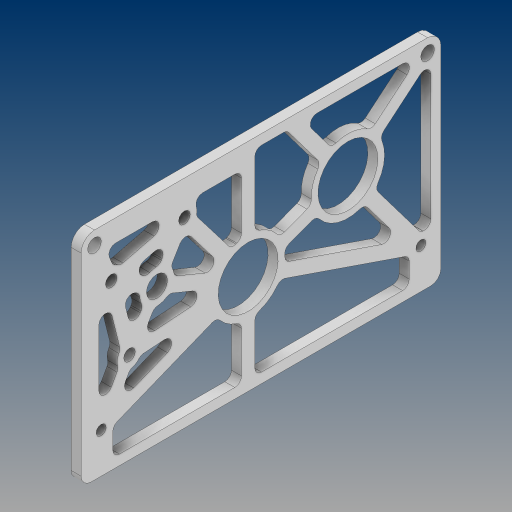
# Autodesk Inventor part: Intake Pivot Gearbox
Saved by Autodesk Inventor 2024.3 (Build 283343000, 343)
## iProperties
Created: 2024-08-01
Part Number: Intake Pivot Gearbox
Material: Generic
Document SubType Name: Modeling
Designer: Kenji
Density: 1 g/cm^3
Appearance: Default
Author: Kenji
Autodesk Inventor part; units mm, degrees
ref_plane "YZ Plane" through (0, 0, 0) normal (1, 0, 0) x (0, 1, 0)
ref_plane "XZ Plane" through (0, 0, 0) normal (0, 1, 0) x (-1, 0, 0)
ref_plane "XY Plane" through (0, 0, 0) normal (0, 0, 1) x (1, 0, 0)
sketch "Sketch1" plane through (0, 0, 0) normal (1, 0, 0) x (0, 1, 0)
  circle A0 centre (65.1002, 0) radius 14.2875
  circle A1 centre (65.1002, 0) radius 31.115 construction
  circle A2 centre (65.1002, 91.0292) radius 10.16 construction
  circle A3 centre (47.2513, 47.5611) radius 36.83 construction
  circle A4 centre (47.2513, 47.5611) radius 15.24 construction
  circle A5 centre (65.1002, 0) radius 35.56 construction
  circle A6 centre (65.1002, 91.0292) radius 30 construction
  circle A7 centre (65.1002, 91.0292) radius 25.4 construction
  circle A8 centre (47.2513, 47.5611) radius 14.2875
  circle A9 centre (47.2513, 47.5611) radius 7.62 construction
  circle A10 centre (19.05, -34.7726) radius 2.3812
  circle A11 centre (19.05, 117.6274) radius 2.3876
  circle A12 centre (47.2513, 47.5611) radius 38.1 construction
  circle A13 centre (65.1002, 0) radius 36.83 construction
  circle A14 centre (96.8502, 120.8024) radius 6.35 construction
  circle A15 centre (96.8502, -37.9476) radius 6.35 construction
  line L0 (92.7754, -33.0774) -> (88.7339, -28.247) construction
  line L1 (103.2002, 120.8024) -> (103.2002, -37.9476)
  circle A16 centre (96.8502, 120.8024) radius 3.2512
  circle A17 centre (96.8502, -37.9476) radius 3.2512
  line L2 (0, 127.1524) -> (0, 108.1024) construction
  line L3 (0, 108.1024) -> (28.575, 108.1024) construction
  line L4 (28.575, 108.1024) -> (28.575, 127.1524) construction
  line L5 (28.575, -25.2476) -> (0, -25.2476) construction
  line L6 (0, -25.2476) -> (0, -44.2976) construction
  line L7 (28.575, -44.2976) -> (28.575, -25.2476) construction
  line L8 (28.575, 127.1524) -> (96.8502, 127.1524)
  line L9 (96.8502, -44.2976) -> (28.575, -44.2976)
  line L10 (0, 122.3772) -> (0, -39.5224)
  arc A18 (96.8502, -44.2976) -> (103.2002, -37.9476) centre (96.8502, -37.9476) ccw
  arc A19 (103.2002, 120.8024) -> (96.8502, 127.1524) centre (96.8502, 120.8024) ccw
  line L11 (28.575, 127.1524) -> (4.7752, 127.1524)
  line L12 (28.575, -44.2976) -> (4.7752, -44.2976)
  arc A20 (28.575, -44.2976) -> (28.575, -44.2976) centre (28.575, -39.5224) ccw
  arc A21 (4.7752, 127.1524) -> (0, 122.3772) centre (4.7752, 122.3772) ccw
  arc A22 (0, -39.5224) -> (4.7752, -44.2976) centre (4.7752, -39.5224) ccw
  circle A23 centre (47.2513, 47.5611) radius 16.51 construction
  line L13 (90.5002, 91.0292) -> (65.1002, 91.0292) construction
  line L14 (92.2182, 116.4588) -> (86.9837, 111.5502) construction
  line L15 (65.1002, 91.0292) -> (89.7457, 97.174) construction
  circle A24 centre (89.7457, 97.174) radius 2.75 construction
  circle A25 centre (78.1822, 112.8012) radius 2.75
  circle A26 centre (58.9554, 115.6747) radius 2.75 construction
  circle A27 centre (43.3282, 104.1111) radius 2.75
  circle A28 centre (40.4547, 84.8843) radius 2.75 construction
  circle A29 centre (52.0182, 69.2571) radius 2.75 construction
  circle A30 centre (71.245, 66.3837) radius 2.75 construction
  circle A31 centre (86.8722, 77.9472) radius 2.75
  circle A32 centre (65.1002, 91.0292) radius 5
  circle A33 centre (65.1002, 0) radius 9.525 construction
  line L16 (103.2002, 0) -> (101.9302, 0) construction
  point P0 (0, 0)
  point P1 (28.575, 117.6274)
  point P2 (33.3502, 127.1524)
  dimension "d10" = 60
  dimension "d0" = 28.575
  dimension "d1" = 65.1002
  dimension "d2" = 62.23
  dimension "d6" = 20.32
  dimension "d7" = 73.66
  dimension "d8" = 30.48
  dimension "d9" = 71.12
  dimension "d11" = 50.8
  dimension "d17" = 28.575
  dimension "d18" = 15.24
  dimension "d20" = 4.7625
  dimension "d22" = 4.7752
  dimension "d24" = 19.05
  dimension "d31" = 12.7
  dimension "d32" = 12.7
  dimension "d35" = 6.5024
  dimension "d36" = 6.5024
  dimension "d37" = 19.05
  dimension "d38" = 9.525
  dimension "d39" = 9.525
  dimension "d40" = 9.525
  dimension "d43" = 4.7752
  dimension "d45" = 4.7752
  dimension "d46" = 4.7752
  dimension "d47" = 1.27
  dimension "d48" = 117.6274
  dimension "d49" = 152.4
  dimension "d52" = 1.27
  dimension "d57" = 14
  dimension "d58" = 5.5
  dimension "d61" = 360
  dimension "d63" = 10
  dimension "d64" = 47.2513
  dimension "d151" = 19.05
  dimension "d152" = 28.575
  dimension "d153" = 19.05
  dimension "d162" = 1.27
  dimension "d163" = 1.27
  constraints: 34 end point, 33 centre point, 20 point on circle, 17 coincident, 16 point on line, 13 tangent, 7 horizontal, 5 vertical alignment, 2 collinear, 2 horizontal alignment, 2 parallel, 2 perpendicular, 1 concentric, 1 midpoint, 1 vertical, 20 other
  measures "d0" diameter of A0
  measures "d1" distance of point (0, 0) A0.centre
  measures "d2" diameter of A1
  measures "d6" diameter of A2
  measures "d7" diameter of A3
  measures "d8" diameter of A4
  measures "d9" diameter of A5
  measures "d11" diameter of A7
  measures "d17" diameter of A8
  measures "d18" diameter of A9
  measures "d20" diameter of A10
  measures "d22" diameter of A11
  measures "d24" horizontal distance of point (0, 0) A10.centre
  measures "d31" diameter of A14
  measures "d32" diameter of A15
  measures "d35" diameter of A16
  measures "d36" diameter of A17
  measures "d37" distance of L2.end L2.start
  measures "d38" distance from line of L3 A11.centre
  measures "d39" distance of A11.centre point (28.575, 117.627)
  measures "d40" distance from line of L5 A10.centre
  measures "d43" radius of A20
  measures "d45" radius of A21
  measures "d46" radius of A22
  measures "d47" radial gap between concentric circles of A3 A12
  measures "d48" vertical distance of A11.centre point (0, 0)
  measures "d49" distance of A10.centre A11.centre
  measures "d52" radial gap between concentric circles of A4 A23
  measures "d57" angle of L13 L15
  measures "d58" diameter of A24
  measures "d63" diameter of A32
  measures "d64" distance from line of L10 A3.centre
  measures "d151" distance of L7.start L5.start
  measures "d152" distance of L5.end L5.start
  measures "d153" diameter of A33
  measures "d162" radial gap between concentric circles of A5 A13
  measures "d163" distance of L16.end L16.start
extrude "Extrusion2" add sketch "Sketch1" along normal blind 4.7625 contours A20 | L1 A18 L9 L12 A22 L10 A21 L11 L8 A19
sketch "Sketch2" plane through (4.7625, 0, 0) normal (1, 0, 0) x (0, 0, -1)
  arc A0 (-127.1524, 4.7752) -> (-122.3772, 0) centre (-122.3772, 4.7752) ccw projected
  line L0 (-122.3772, 0) -> (39.5224, 0) projected
  arc A1 (39.5224, 0) -> (44.2976, 4.7752) centre (39.5224, 4.7752) ccw projected
  line L1 (44.2976, 4.7752) -> (44.2976, 96.8502) projected
  arc A2 (44.2976, 96.8502) -> (37.9476, 103.2002) centre (37.9476, 96.8502) ccw projected
  line L2 (37.9476, 103.2002) -> (-120.8024, 103.2002) projected
  arc A3 (-120.8024, 103.2002) -> (-127.1524, 96.8502) centre (-120.8024, 96.8502) ccw projected
  line L3 (-127.1524, 96.8502) -> (-127.1524, 4.7752) projected
  circle A4 centre (-91.0292, 65.1002) radius 5 projected
  circle A5 centre (0, 65.1002) radius 14.2875 projected
  circle A6 centre (-47.5611, 47.2513) radius 14.2875 projected
  circle A7 centre (34.7726, 19.05) radius 2.3812 projected
  circle A8 centre (-117.6274, 19.05) radius 2.3876 projected
  circle A9 centre (-112.8012, 78.1822) radius 2.75 projected
  circle A10 centre (-104.1111, 43.3282) radius 2.75 projected
  circle A11 centre (-77.9472, 86.8722) radius 2.75 projected
  circle A12 centre (37.9476, 96.8502) radius 3.2512 projected
  circle A13 centre (-120.8024, 96.8502) radius 3.2512 projected
  circle A14 centre (-77.9472, 86.8722) radius 5.925 construction
  circle A15 centre (-47.5611, 47.2513) radius 17.4625 construction
  circle A16 centre (0, 65.1002) radius 17.4625 construction
  circle A17 centre (-91.0292, 65.1002) radius 8.175 construction
  circle A18 centre (-112.8012, 78.1822) radius 5.925 construction
  circle A19 centre (-104.1111, 43.3282) radius 5.925 construction
  circle A20 centre (-117.6274, 19.05) radius 5.5626 construction
  circle A21 centre (34.7726, 19.05) radius 5.5562 construction
  circle A22 centre (37.9476, 96.8502) radius 6.4262 construction
  circle A23 centre (-120.8024, 96.8502) radius 6.4262 construction
  line L4 (-107.7225, 75.1306) -> (-98.0365, 69.3106) construction
  line L5 (-86.8187, 72.1075) -> (-80.9988, 81.7935) construction
  line L6 (-83.4669, 61.995) -> (-63.7148, 53.8843) construction
  line L7 (-95.2396, 58.0929) -> (-101.0595, 48.4069) construction
  line L8 (-31.0408, 41.5927) -> (29.5162, 20.8505) construction
  line L9 (-31.212, 53.3868) -> (-16.3491, 58.9646) construction
  line L10 (-63.7606, 40.731) -> (-112.4671, 21.127) construction
  line L11 (13.393, 76.3059) -> (33.019, 92.7265) construction
  line L12 (-58.188, 61.1079) -> (-74.3415, 82.1707) construction
  line L13 (31.4244, 23.4841) -> (10.5229, 51.1644) construction
  line L14 (-83.6962, 85.4389) -> (-107.0522, 79.6156) construction
  line L15 (-111.3678, 72.4332) -> (-105.5445, 49.0772) construction
  line L16 (-106.9932, 38.1513) -> (-114.9216, 23.9102) construction
  line L17 (-98.2003, 43.7382) -> (-64.9817, 46.0427) construction
  line L18 (-47.5611, 29.7888) -> (-47.5611, 4.7752) construction
  line L19 (-30.2923, 57.1232) -> (-19.4999, 61.1734)
  line L20 (13.0228, 80.1359) -> (28.1768, 92.8149)
  line L21 (33.6952, 25.7457) -> (14.3667, 51.3429)
  line L22 (17.0976, 75.2657) -> (34.4618, 89.794)
  line L23 (19.7368, 33.6934) -> (9.2991, 47.5164)
  line L24 (-27.9555, 43.892) -> (16.1742, 28.7765)
  line L25 (-30.0131, 37.8846) -> (27.0702, 18.3322)
  line L26 (-28.0612, 51.178) -> (-17.2688, 55.2283)
  arc A24 (-13.6681, 54.2318) -> (5.7245, 48.6027) centre (0, 65.1002) ccw
  arc A25 (-30.1012, 46.9504) -> (-30.1172, 48.0587) centre (-47.5611, 47.2513) ccw
  arc A26 (-13.6681, 54.2318) -> (-17.2688, 55.2283) centre (-16.1532, 52.2557) ccw
  arc A27 (9.2991, 47.5164) -> (5.7245, 48.6027) centre (6.7653, 45.6031) ccw
  arc A28 (-28.0612, 51.178) -> (-30.1172, 48.0587) centre (-26.9456, 48.2055) ccw
  arc A29 (-30.1012, 46.9504) -> (-27.9555, 43.892) centre (-26.9266, 46.8956) ccw
  arc A30 (16.1742, 28.7765) -> (19.7368, 33.6934) centre (17.203, 31.7802) ccw
  line L27 (-44.3861, 27.615) -> (-44.3861, 7.9502)
  line L28 (-50.7361, 27.615) -> (-50.7361, 7.9502)
  line L29 (-41.2111, 4.7752) -> (26.0414, 4.7752)
  arc A31 (-42.188, 30.6359) -> (-33.5834, 36.784) centre (-47.5611, 47.2513) ccw
  arc A32 (-30.0131, 37.8846) -> (-33.5834, 36.784) centre (-31.042, 34.8809) ccw
  arc A33 (-42.188, 30.6359) -> (-44.3861, 27.615) centre (-41.2111, 27.615) ccw
  arc A34 (-44.3861, 7.9502) -> (-41.2111, 4.7752) centre (-41.2111, 7.9502) ccw
  line L30 (39.5224, 87.3833) -> (39.5224, 27.6381)
  arc A35 (36.9782, 90.4975) -> (36.8766, 90.5139) centre (37.9476, 96.8502) ccw
  arc A36 (14.3004, 55.0783) -> (16.1911, 71.6413) centre (0, 65.1002) ccw
  arc A37 (35.7747, 24.5151) -> (35.6994, 24.5284) centre (34.7726, 19.05) ccw
  arc A38 (35.7747, 24.5151) -> (39.5224, 27.6381) centre (36.3474, 27.6381) ccw
  arc A39 (33.6952, 25.7457) -> (35.6994, 24.5284) centre (36.229, 27.6589) ccw
  arc A40 (39.5224, 87.3833) -> (36.8766, 90.5139) centre (36.3474, 87.3833) ccw
  arc A41 (36.9782, 90.4975) -> (34.4618, 89.794) centre (36.4992, 87.3589) ccw
  arc A42 (17.0976, 75.2657) -> (16.1911, 71.6413) centre (19.135, 72.8306) ccw
  arc A43 (14.3004, 55.0783) -> (14.3667, 51.3429) centre (16.9004, 53.2562) ccw
  line L31 (-47.5611, 64.7138) -> (-47.5611, 98.425) construction
  line L32 (-44.3861, 66.8875) -> (-44.3861, 95.25)
  line L33 (-50.7361, 66.8875) -> (-50.7361, 89.6222)
  line L34 (-41.2111, 98.425) -> (-30.7232, 98.425)
  arc A44 (-41.2111, 98.425) -> (-44.3861, 95.25) centre (-41.2111, 95.25) ccw
  arc A45 (31.7173, 98.425) -> (31.6252, 95.7001) centre (37.9476, 96.8502) ccw
  arc A46 (28.1768, 92.8149) -> (26.1394, 98.425) centre (26.1394, 95.25) ccw
  arc A47 (9.2954, 79.8831) -> (13.0228, 80.1359) centre (10.9854, 82.5709) ccw
  arc A48 (-33.893, 58.1197) -> (-42.188, 63.8666) centre (-47.5611, 47.2513) ccw
  arc A49 (-44.3861, 66.8875) -> (-42.188, 63.8666) centre (-41.2111, 66.8875) ccw
  arc A50 (-33.893, 58.1197) -> (-30.2923, 57.1232) centre (-31.4079, 60.0957) ccw
  line L35 (-53.9111, 4.7752) -> (-108.8898, 4.7752)
  line L36 (-112.0648, 15.7218) -> (-112.0648, 7.9502)
  line L37 (-64.5917, 36.974) -> (-110.0753, 18.6671)
  arc A51 (-60.9685, 36.0629) -> (-52.9341, 30.6359) centre (-47.5611, 47.2513) ccw
  arc A52 (-60.9685, 36.0629) -> (-64.5917, 36.974) centre (-63.4062, 34.0286) ccw
  arc A53 (-50.7361, 27.615) -> (-52.9341, 30.6359) centre (-53.9111, 27.615) ccw
  arc A54 (-53.9111, 4.7752) -> (-50.7361, 7.9502) centre (-53.9111, 7.9502) ccw
  arc A55 (-112.0648, 7.9502) -> (-108.8898, 4.7752) centre (-108.8898, 7.9502) ccw
  line L38 (-86.032, 35.1895) -> (-102.164, 28.6965)
  line L39 (-104.5077, 36.0886) -> (-106.1235, 33.1862)
  line L40 (-97.3888, 40.6119) -> (-87.4372, 41.3023)
  arc A56 (-102.5631, 37.6089) -> (-99.5911, 39.4973) centre (-104.1111, 43.3282) ccw
  arc A57 (-86.032, 35.1895) -> (-87.4372, 41.3023) centre (-87.2174, 38.1349) ccw
  arc A58 (-106.1235, 33.1862) -> (-102.164, 28.6965) centre (-103.3494, 31.6418) ccw
  arc A59 (-97.3888, 40.6119) -> (-99.5911, 39.4973) centre (-97.169, 37.4445) ccw
  arc A60 (-102.5631, 37.6089) -> (-104.5077, 36.0886) centre (-101.7336, 34.5442) ccw
  line L41 (-56.9915, 64.765) -> (-71.4611, 83.6321)
  line L42 (-53.9111, 92.7972) -> (-69.2727, 92.7972)
  arc A61 (-72.0837, 86.0206) -> (-72.2992, 88.6628) centre (-77.9472, 86.8722) ccw
  arc A62 (-69.2727, 92.7972) -> (-72.2992, 88.6628) centre (-69.2727, 89.6222) ccw
  arc A63 (-72.0837, 86.0206) -> (-71.4611, 83.6321) centre (-68.9417, 85.5643) ccw
  arc A64 (-50.7361, 89.6222) -> (-53.9111, 92.7972) centre (-53.9111, 89.6222) ccw
  arc A65 (-52.9341, 63.8666) -> (-53.4089, 63.7055) centre (-47.5611, 47.2513) ccw
  arc A66 (-56.9915, 64.765) -> (-53.4089, 63.7055) centre (-54.4721, 66.6972) ccw
  arc A67 (-52.9341, 63.8666) -> (-50.7361, 66.8875) centre (-53.9111, 66.8875) ccw
  line L43 (-64.407, 63.9998) -> (-74.7895, 77.5376)
  line L44 (-83.4625, 71.5287) -> (-80.0304, 77.2407)
  line L45 (-81.1208, 64.4639) -> (-68.1324, 59.1306)
  arc A68 (-74.7895, 77.5376) -> (-80.0304, 77.2407) centre (-77.3089, 75.6054) ccw
  arc A69 (-83.0239, 66.7573) -> (-83.6189, 68.5526) centre (-91.0292, 65.1002) ccw
  arc A70 (-83.4625, 71.5287) -> (-83.6189, 68.5526) centre (-80.741, 69.8935) ccw
  arc A71 (-83.0239, 66.7573) -> (-81.1208, 64.4639) centre (-79.9148, 67.4009) ccw
  arc A72 (-68.1324, 59.1306) -> (-64.407, 63.9998) centre (-66.9264, 62.0676) ccw
  line L46 (-83.5328, 58.5898) -> (-73.9173, 54.6414)
  line L47 (-93.1529, 55.4012) -> (-95.1113, 52.1418)
  line L48 (-92.17, 47.3392) -> (-74.9036, 48.537)
  arc A73 (-90.5986, 56.9365) -> (-86.4985, 58.2955) centre (-91.0292, 65.1002) ccw
  arc A74 (-83.5328, 58.5898) -> (-86.4985, 58.2955) centre (-84.7388, 55.6528) ccw
  arc A75 (-90.5986, 56.9365) -> (-93.1529, 55.4012) centre (-90.4313, 53.766) ccw
  arc A76 (-95.1113, 52.1418) -> (-92.17, 47.3392) centre (-92.3898, 50.5066) ccw
  arc A77 (-74.9036, 48.537) -> (-73.9173, 54.6414) centre (-75.1233, 51.7044) ccw
  line L49 (-112.4705, 63.7318) -> (-108.7687, 48.8847)
  line L50 (-110.0558, 39.1774) -> (-112.7771, 34.2893)
  arc A78 (-109.1495, 46.4459) -> (-109.7879, 41.6312) centre (-104.1111, 43.3282) ccw
  arc A79 (-109.1495, 46.4459) -> (-108.7687, 48.8847) centre (-111.8494, 48.1166) ccw
  arc A80 (-110.0558, 39.1774) -> (-109.7879, 41.6312) centre (-112.8299, 40.7218) ccw
  line L51 (-92.054, 80.0828) -> (-97.1582, 78.8102)
  line L52 (-88.9055, 74.7992) -> (-88.5644, 75.3669)
  line L53 (-98.0254, 73.008) -> (-97.4577, 72.6669)
  arc A81 (-91.4598, 73.2639) -> (-94.4816, 72.5104) centre (-91.0292, 65.1002) ccw
  arc A82 (-97.4577, 72.6669) -> (-94.4816, 72.5104) centre (-95.8224, 75.3884) ccw
  arc A83 (-91.4598, 73.2639) -> (-88.9055, 74.7992) centre (-91.627, 76.4344) ccw
  arc A84 (-88.5644, 75.3669) -> (-92.054, 80.0828) centre (-91.2859, 77.0021) ccw
  arc A85 (-97.1582, 78.8102) -> (-98.0254, 73.008) centre (-96.3901, 75.7295) ccw
  line L54 (-101.2959, 67.565) -> (-100.7282, 67.2239)
  line L55 (-106.0118, 64.0754) -> (-104.7392, 58.9711)
  line L56 (-98.5959, 58.6717) -> (-98.937, 58.104)
  arc A86 (-99.1928, 64.6696) -> (-98.4394, 61.6478) centre (-91.0292, 65.1002) ccw
  arc A87 (-101.2959, 67.565) -> (-106.0118, 64.0754) centre (-102.9311, 64.8435) ccw
  arc A88 (-99.1928, 64.6696) -> (-100.7282, 67.2239) centre (-102.3634, 64.5024) ccw
  arc A89 (-98.5959, 58.6717) -> (-98.4394, 61.6478) centre (-101.3174, 60.3069) ccw
  arc A90 (-104.7392, 58.9711) -> (-98.937, 58.104) centre (-101.6585, 59.7392) ccw
  line L57 (-92.3976, 86.5416) -> (-107.2447, 82.8398)
  line L58 (-118.2708, 90.9437) -> (-115.1353, 83.628) construction
  line L59 (-93.1657, 92.7972) -> (-110.7958, 92.7972)
  line L60 (-113.7141, 88.3715) -> (-112.4508, 85.4241)
  arc A91 (-109.6835, 83.2206) -> (-110.673, 83.7117) centre (-112.8012, 78.1822) ccw
  arc A92 (-92.3976, 86.5416) -> (-93.1657, 92.7972) centre (-93.1657, 89.6222) ccw
  arc A93 (-112.4508, 85.4241) -> (-110.673, 83.7117) centre (-109.5325, 86.6749) ccw
  arc A94 (-109.6835, 83.2206) -> (-107.2447, 82.8398) centre (-108.0128, 85.9205) ccw
  line L61 (-10.5229, 79.036) -> (-25.1636, 98.425) construction
  line L62 (-14.3667, 78.8575) -> (-28.1894, 97.1633)
  line L63 (-9.2991, 82.684) -> (-17.343, 93.3367)
  arc A95 (-28.1894, 97.1633) -> (-30.7232, 98.425) centre (-30.7232, 95.25) ccw
  line L64 (-14.8092, 98.425) -> (26.1394, 98.425)
  arc A96 (-14.8092, 98.425) -> (-17.343, 93.3367) centre (-14.8092, 95.25) ccw
  arc A97 (9.2954, 79.8831) -> (-5.7245, 81.5977) centre (0, 65.1002) ccw
  arc A98 (-14.3004, 75.1221) -> (-17.4438, 64.2928) centre (0, 65.1002) ccw
  arc A99 (-14.3004, 75.1221) -> (-14.3667, 78.8575) centre (-16.9004, 76.9442) ccw
  arc A100 (-19.4999, 61.1734) -> (-17.4438, 64.2928) centre (-20.6154, 64.146) ccw
  arc A101 (-9.2991, 82.684) -> (-5.7245, 81.5977) centre (-6.7653, 84.5973) ccw
  line L65 (29.2164, 7.9502) -> (29.2164, 15.3285)
  arc A102 (29.2164, 15.3285) -> (27.0702, 18.3322) centre (26.0414, 15.3285) ccw
  arc A103 (26.0414, 4.7752) -> (29.2164, 7.9502) centre (26.0414, 7.9502) ccw
  arc A104 (-110.0753, 18.6671) -> (-112.0648, 15.7218) centre (-108.8898, 15.7218) ccw
  arc A105 (-110.7958, 92.7972) -> (-113.7141, 88.3715) centre (-110.7958, 89.6222) ccw
  line L66 (-118.7262, 35.8337) -> (-118.7262, 62.9637)
  arc A106 (-118.7262, 35.8337) -> (-112.7771, 34.2893) centre (-115.5512, 35.8337) ccw
  arc A107 (-112.4705, 63.7318) -> (-118.7262, 62.9637) centre (-115.5512, 62.9637) ccw
  point P0 (0, 0)
  point P1 (-112.0648, 4.7752)
  point P2 (-32.6, 56.2571)
  point P3 (-17.1922, 62.0395)
  point P4 (11.1324, 78.5542)
  point P5 (34.5587, 24.6021)
  point P6 (12.8813, 53.3099)
  point P7 (15.2072, 73.684)
  point P8 (35.6999, 90.8299)
  point P9 (7.8138, 49.4834)
  point P10 (-30.2873, 44.6907)
  point P11 (-32.345, 38.6833)
  point P12 (29.4301, 17.5239)
  point P13 (-30.3689, 50.312)
  point P14 (-14.9611, 56.0943)
  point P15 (-44.3861, 30.0798)
  point P16 (-50.7361, 30.0798)
  point P17 (-50.7361, 4.7752)
  point P18 (39.5224, 90.6199)
  point P19 (39.5224, 21.9329)
  point P20 (-44.3861, 64.4227)
  point P21 (-44.3861, 98.425)
  point P22 (-50.7361, 64.4227)
  point P23 (-112.0648, 19.05)
  point P24 (-62.3051, 37.8943)
  point P25 (-112.2048, 17.8101)
  point P26 (-112.0648, 17.8664)
  point P27 (-103.7704, 37.413)
  point P28 (-98.9009, 40.507)
  point P29 (-55.4915, 62.8091)
  point P30 (-72.3835, 84.8349)
  point P31 (-77.9472, 92.7972)
  point P32 (-77.4223, 80.9705)
  point P33 (-84.4277, 69.9222)
  point P34 (-77.8022, 80.949)
  point P35 (-82.8545, 65.1758)
  point P36 (-85.2665, 59.3017)
  point P37 (-64.6515, 50.8367)
  point P38 (-92.1876, 57.0077)
  point P39 (-108.402, 47.414)
  point P40 (-109.3185, 40.5017)
  point P41 (-118.1797, 24.5851)
  point P42 (-114.6717, 72.5602)
  point P43 (-118.1797, 24.5851)
  point P44 (-89.8708, 73.1927)
  point P45 (-95.8512, 71.7016)
  point P46 (-99.1217, 66.2586)
  point P47 (-97.6306, 60.2782)
  point P48 (-108.7154, 82.4731)
  point P49 (-115.8155, 92.7972)
  point P50 (-115.6832, 92.9657)
  point P51 (-111.8537, 84.0309)
  point P52 (-115.6832, 92.9657)
  point P53 (-12.8813, 76.8905)
  point P54 (-7.8138, 80.717)
  point P55 (-21.1851, 98.425)
  point P56 (-17.1922, 62.0395)
  point P57 (-114.6717, 72.5602)
  point P58 (36.9272, 90.5049)
  point P59 (-118.7262, 24.503)
  dimension "d68" = 3.175
  dimension "d69" = 3.175
  dimension "d70" = 3.175
  dimension "d71" = 3.175
  dimension "d72" = 3.175
  dimension "d73" = 3.175
  dimension "d74" = 3.175
  dimension "d75" = 3.175
  dimension "d76" = 3.175
  dimension "d77" = 3.175
  dimension "d78" = 3.175
  dimension "d79" = 3.175
  dimension "d80" = 3.175
  dimension "d81" = 3.175
  dimension "d82" = 3.175
  dimension "d83" = 3.175
  dimension "d84" = 3.175
  dimension "d85" = 3.175
  dimension "d86" = 3.175
  dimension "d87" = 3.175
  dimension "d88" = 3.175
  dimension "d90" = 4.7752
  dimension "d91" = 3.175
  dimension "d95" = 4.7752
  dimension "d96" = 3.175
  dimension "d97" = 3.175
  dimension "d98" = 3.175
  dimension "d99" = 3.175
  dimension "d100" = 3.175
  dimension "d101" = 3.175
  dimension "d102" = 3.175
  dimension "d104" = 3.175
  dimension "d105" = 3.175
  dimension "d106" = 3.175
  dimension "d107" = 3.175
  dimension "d108" = 3.175
  dimension "d109" = 3.175
  dimension "d110" = 3.175
  dimension "d111" = 4.7752
  dimension "d112" = 3.175
  dimension "d113" = 3.175
  dimension "d114" = 3.175
  dimension "d115" = 3.175
  dimension "d116" = 3.175
  dimension "d117" = 3.175
  dimension "d118" = 3.175
  dimension "d119" = 3.175
  dimension "d120" = 3.175
  dimension "d121" = 3.175
  dimension "d122" = 3.175
  dimension "d123" = 3.175
  dimension "d124" = 3.175
  dimension "d125" = 3.175
  dimension "d128" = 3.175
  dimension "d129" = 3.175
  dimension "d131" = 3.175
  dimension "d132" = 3.175
  dimension "d133" = 3.175
  dimension "d134" = 3.175
  dimension "d135" = 3.175
  dimension "d136" = 3.175
  dimension "d137" = 3.175
  dimension "d138" = 3.175
  dimension "d139" = 3.175
  constraints: 217 point on circle, 129 tangent, 126 end point, 104 point on line, 87 centre point, 35 equal radius, 35 parallel, 7 vertical, 4 concentric, 4 horizontal, 3 perpendicular, 2 collinear, 105 other
  measures "d75" radial gap between concentric circles of A7 A21
  measures "d76" radial gap between concentric circles of A12 A22
  measures "d77" radial gap between concentric circles of A13 A23
  measures "d78" distance between parallel lines of L9 L19
  measures "d79" distance between parallel lines of L11 L20
  measures "d80" distance between parallel lines of L13 L21
  measures "d81" distance between parallel lines of L11 L22
  measures "d82" distance between parallel lines of L13 L23
  measures "d83" distance between parallel lines of L8 L24
  measures "d84" distance between parallel lines of L8 L25
  measures "d85" distance between parallel lines of L9 L26
  measures "d86" radius of A26
  measures "d87" distance between parallel lines of L18 L27
  measures "d88" distance between parallel lines of L18 L28
  measures "d90" distance between parallel lines of L0 L29
  measures "d91" radius of A32
  measures "d95" distance between parallel lines of L1 L30
  measures "d96" radius of A38
  measures "d97" distance between parallel lines of L31 L32
  measures "d98" distance between parallel lines of L31 L33
  measures "d99" radius of A44
  measures "d100" radius of A46
  measures "d101" radius of A47
  measures "d102" radius of A49
  measures "d104" distance between parallel lines of L10 L37
  measures "d105" radius of A52
  measures "d106" distance between parallel lines of L10 L38
  measures "d107" distance between parallel lines of L16 L39
  measures "d108" distance between parallel lines of L17 L40
  measures "d109" radius of A57
  measures "d110" distance between parallel lines of L12 L41
  measures "d111" distance between parallel lines of L34 L2
  measures "d112" radius of A62
  measures "d113" radius of A66
  measures "d114" distance between parallel lines of L12 L43
  measures "d115" distance between parallel lines of L5 L44
  measures "d116" distance between parallel lines of L6 L45
  measures "d117" radius of A68
  measures "d118" radius of A70
  measures "d119" distance between parallel lines of L6 L46
  measures "d120" distance between parallel lines of L7 L47
  measures "d121" distance between parallel lines of L17 L48
  measures "d122" radius of A74
  measures "d123" radius of A77
  measures "d124" distance between parallel lines of L15 L49
  measures "d125" distance between parallel lines of L16 L50
  measures "d128" radius of A79
  measures "d129" radius of A80
  measures "d131" distance between parallel lines of L14 L51
  measures "d132" distance between parallel lines of L5 L52
  measures "d133" distance between parallel lines of L4 L53
  measures "d134" radius of A82
  measures "d135" distance between parallel lines of L4 L54
  measures "d136" distance between parallel lines of L15 L55
  measures "d137" distance between parallel lines of L7 L56
  measures "d138" radius of A87
  measures "d139" distance between parallel lines of L14 L57
extrude "Extrusion3" cut sketch "Sketch2" against normal blind 4.7625 contours A40 L30 A38 A37 A39 L21 A43 A36 A42 L22 A41 | A50 A48 A49 L32 A44 L34 A95 L62 A99 A98 A100 L19 | A47 A97 A101 L63 A96 L64 A46 L20 | A30 L24 A29 A25 A28 L26 A26 A24 A27 L23 | L25 A102 L65 A103 L29 A34 L27 A33 A31 A32 | L28 A54 L35 A55 L36 A104 L37 A52 A51 A53 | A67 A65 A66 L41 A63 A61 A62 L42 A64 L33 | L38 A58 L39 A60 A56 A59 L40 A57 | A72 L45 A71 A69 A70 L44 A68 L43 | L46 A77 L48 A76 L47 A75 A73 A74 | L49 A79 A78 A80 L50 A106 L66 A107 | A84 L52 A83 A81 A82 L53 A85 L51 | L54 A88 A86 A89 L56 A90 L55 A87 | L57 A94 A91 A93 L60 A105 L59 A92
body "Solid2"
